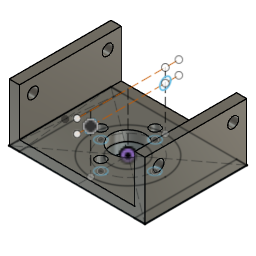
lab1-link90 v4 (Autodesk Fusion 360 design; units mm, degrees)
Autodesk Fusion 360 part; units mm, degrees
sketch "Sketch1" plane through (0, 0, 0) normal (0, 0, 1) x (1, 0, 0)
  line L0 (20, 15) -> (-20, 15)
  line L1 (-20, 15) -> (-20, -15)
  line L2 (-20, -15) -> (20, -15)
  line L3 (20, -15) -> (20, 15)
  line L4 (20, 15) -> (-20, -15) construction
  line L5 (-20, 15) -> (20, -15) construction
  circle A0 centre (0, 0) radius 11
  circle A1 centre (0, 0) radius 8 construction
  circle A2 centre (0, 0) radius 5
  circle A3 centre (0, 8) radius 1.5
  circle A4 centre (0, -8) radius 1.5
  circle A5 centre (7.9991, -0.1196) radius 1.5
  circle A6 centre (-8, 0) radius 1.5
  line L6 (-20, 15) -> (-17, 15)
  line L7 (-17, 15) -> (-17, -15)
  line L8 (-17, -15) -> (-20, -15)
  line L9 (-20, -15) -> (-20, 15)
  line L10 (-20, 15) -> (-17, -15) construction
  line L11 (-17, 15) -> (-20, -15) construction
  line L12 (0, 15) -> (0, -15) construction
  line L13 (20, -15) -> (20, 15)
  line L14 (17, 15) -> (17, -15)
  line L15 (17, -15) -> (20, -15)
  line L16 (20, 15) -> (17, 15)
  point P0 (-18.5, 0)
  dimension "d1" = 40
  dimension "d2" = 30
  dimension "d3" = 22
  dimension "d4" = 16
  dimension "d5" = 10
  dimension "d6" = 3
  dimension "d7" = 3
  dimension "d9" = 3
  dimension "d10" = 3
  dimension "d11" = 30
  dimension "d12" = 3
  constraint horizontal L0
  constraint perpendicular L0 L1
  constraint parallel L0 L2
  constraint parallel L1 L3
  constraint coincident L4 A0.centre
  constraint coincident L5 A0.centre
  constraint coincident A0.centre A1.centre
  constraint concentric A1 A2
  constraint coincident A1 A3.centre
  constraint coincident A1 A4.centre
  constraint coincident A1 A5.centre
  constraint coincident A1 A6.centre
  constraint horizontal L6
  constraint perpendicular L6 L7
  constraint parallel L6 L8
  constraint parallel L7 L9
  constraint coincident L10 P0
  constraint coincident L11 P0
  constraint midpoint L0 L12.start
  constraint midpoint L2 L12.end
  constraint symmetric L0.end L12 L0.start
  constraint symmetric L6.end L12 L14.start
  constraint symmetric L7.end L12 L14.end
  constraint symmetric L1.end L12 L2.end
  measures "d1" distance of L0.start L0.end
  measures "d2" distance of L0.start L2.end
  measures "d3" diameter of A0
  measures "d4" diameter of A1
  measures "d5" diameter of A2
  measures "d6" diameter of A3
  measures "d7" diameter of A4
  measures "d9" diameter of A5
  measures "d10" diameter of A6
  measures "d11" distance of L0.end L1.end
  measures "d12" distance of L1 L7
extrude "Extrude1" add sketch "Sketch1" along normal blind 3 contours L0 L2 L7 L14
extrude "Extrude2" add sketch "Sketch1" along normal blind 3 contours A0
extrude "Extrude3" add sketch "Sketch1" against normal blind 3 contours A0
extrude "Extrude4" add sketch "Sketch1" along normal blind 17 contours L0 L1 L2 L6 L7 L8 L9
extrude "Extrude5" add sketch "Sketch1" along normal blind 17 contours L0 L2 L3 L13 L14 L15 L16
sketch "Sketch2" plane through (0, 0, 0) normal (1, 0, 0) x (0, 1, 0)
  line L0 (-15, 12.9476) -> (15, 12.9476) construction
  line L1 (-15, 16.9476) -> (15, 16.9476) construction
  line L2 (0, 16.9476) -> (0, 0) construction
  line L3 (-11, 16.9476) -> (-11, 0) construction
  line L4 (11, 16.9476) -> (11, 0) construction
  circle A0 centre (-11, 12.9476) radius 1.6
  circle A1 centre (11, 12.9476) radius 1.6
  dimension "d23" = 4
  dimension "d24" = 11
  dimension "d25" = 3.2
  constraint horizontal L0
  constraint horizontal L1
  constraint midpoint L1 L2.start
  constraint coincident L2.end origin
  constraint coincident L1 L3.start
  constraint perpendicular L0 L3
  constraint vertical L2
  constraint symmetric L2 L3.start L4.start
  constraint symmetric L2 L3.end L4.end
  constraint coincident L0 A0.centre
  constraint coincident L3 A0.centre
  constraint symmetric L2 A0 A1
  measures "d23" distance of L0 L1
  measures "d24" distance of L2 L3
  measures "d25" diameter of A0
extrude "Extrude6" cut sketch "Sketch2" along normal blind 28
extrude "Extrude7" cut sketch "Sketch2" against normal blind 25
